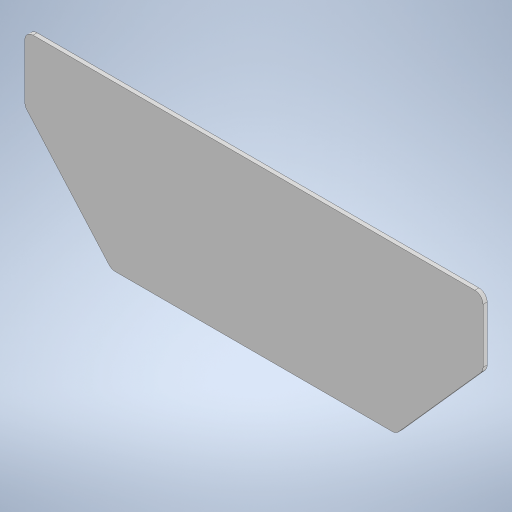
# Autodesk Inventor part: wedge
Saved by Autodesk Inventor 2023.4 (Build 274418000, 418)
## iProperties
Created: 2023-12-11
Part Number: wedge
Material: Generic
Document SubType Name: Modeling
Designer: Meer
Density: 1 g/cm^3
Appearance: Default
Author: Meer
Autodesk Inventor part; units mm, degrees
ref_plane "YZ Plane" through (0, 0, 0) normal (1, 0, 0) x (0, 1, 0)
ref_plane "XZ Plane" through (0, 0, 0) normal (0, 1, 0) x (-1, 0, 0)
ref_plane "XY Plane" through (0, 0, 0) normal (0, 0, 1) x (1, 0, 0)
sketch "Sketch1" plane through (0, 0, 0) normal (0, 0, 1) x (1, 0, 0)
  line L0 (-83.8471, 83.8315) -> (93.9529, 83.8315)
  line L1 (93.9529, 83.8315) -> (93.9529, 20.3315)
  line L2 (93.9529, 20.3315) -> (-83.8471, 20.3315)
  line L3 (-83.8471, 20.3315) -> (-83.8471, 83.8315)
  line L4 (-83.8471, 20.3315) -> (-83.8471, 58.4315)
  line L5 (93.9529, 20.3315) -> (93.9529, 58.2798)
  line L6 (93.9529, 58.2798) -> (60.1807, 20.3315)
  line L7 (-83.8471, 58.4315) -> (-50.246, 20.3315)
  point P0 (0, 0)
  dimension "d0" = 177.8
  dimension "d1" = 63.5
  dimension "d2" = 38.1
  dimension "d3" = 50.8
  dimension "d4" = 50.8
  constraints: 16 end point, 4 point on line, 2 parallel, 1 horizontal, 1 perpendicular
  measures "d0" distance of L0.start L0.end
  measures "d1" distance of L0.end L1.end
  measures "d2" distance of L2.end L4.end
  measures "d3" distance of L5.end L6.end
  measures "d4" distance of L4.end L7.end
extrude "Extrusion1" add sketch "Sketch1" along normal blind 1.5875 contours L0 L1 L6 L2 L7 L3
fillet "Fillet1" radius 3.175 1 edges at (93.9529, 83.8315, 0.7937)
fillet "Fillet2" radius 3.175 1 edges at (93.9529, 58.2798, 0.7937)
fillet "Fillet3" radius 3.175 1 edges at (60.1807, 20.3315, 0.7937)
fillet "Fillet4" radius 3.175 2 edges at (-50.246, 20.3315, 0.7937) (-83.8471, 58.4315, 0.7937)
fillet "Fillet5" radius 3.175 1 edges at (-83.8471, 83.8315, 0.7937)
body "Solid1"
